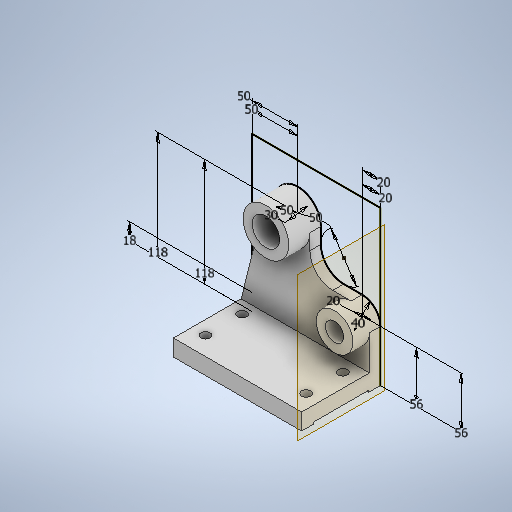
# Autodesk Inventor part: Baitap2
Saved by Autodesk Inventor 2025.2 (Build 292293000, 293)
## iProperties
Created: 2024-12-04
Part Number: Baitap2
Material: Generic
Document SubType Name: Modeling
Designer: hongquan
Density: 1 g/cm^3
Appearance: Default
Author: hongquan
Autodesk Inventor part; units mm, degrees
ref_plane "YZ Plane" through (0, 0, 0) normal (1, 0, 0) x (0, 1, 0)
ref_plane "XZ Plane" through (0, 0, 0) normal (0, 1, 0) x (-1, 0, 0)
ref_plane "XY Plane" through (0, 0, 0) normal (0, 0, 1) x (1, 0, 0)
sketch "Sketch1" plane through (0, 0, 0) normal (1, 0, 0) x (0, 1, 0)
  line L0 (0, 0) -> (168, 0)
  line L1 (168, 0) -> (168, -86)
  line L2 (168, -86) -> (0, -86)
  line L3 (0, -86) -> (0, 0)
  dimension "d0" = 86
  dimension "d1" = 168
  constraints: 8 end point, 2 parallel, 1 horizontal, 1 perpendicular
  measures "d0" distance of L2.end L0.start
  measures "d1" distance of L1.end L2.end
extrude "Extrusion1" add sketch "Sketch1" along normal blind 140
sketch "Sketch2" plane through (140, 0, 0) normal (1, 0, 0) x (0, 0, -1)
  line L0 (0, 0) -> (86, 0) projected
  line L1 (0, 0) -> (0, 2)
  line L2 (13, 2) -> (73, 2)
  line L3 (0, 168) -> (0, 0) projected
  line L4 (86, 168) -> (0, 168) projected
  line L5 (43, 168) -> (43, 0)
  line L6 (13, 2) -> (13, 0)
  line L7 (73, 2) -> (73, 0)
  line L8 (13, 0) -> (73, 0)
  point P0 (43, 2)
  dimension "d5" = 60
  dimension "d6" = 2
  constraints: 12 end point, 4 point on line, 3 midpoint, 2 collinear, 2 perpendicular, 1 horizontal, 1 vertical
  measures "d5" distance of L2.start L2.end
  measures "d6" distance from line of L0 L2.end
extrude "Extrusion2" cut sketch "Sketch2" against normal blind 140 contours L6 L2 L5 L0 | L5 L2 L7 L0
sketch "Sketch3" plane through (0, 0, -86) normal (0, 0, -1) x (-1, 0, 0)
  line L0 (-140, 0) -> (-140, 168) projected
  line L1 (-140, 0) -> (-140, 56)
  circle A0 centre (-120, 56) radius 10
  circle A1 centre (-120, 56) radius 20
  line L2 (0, 0) -> (-140, 0) projected
  circle A2 centre (-50, 118) radius 15
  circle A3 centre (-50, 118) radius 25
  line L3 (0, 0) -> (0, 168) projected
  arc A4 (-100, 76) -> (-75, 101) centre (-100, 101) ccw
  line L4 (0, 18) -> (0, 0)
  line L5 (-25, 118) -> (0, 18)
  line L6 (-75, 101) -> (-75, 118)
  line L7 (-100, 76) -> (-120, 76)
  line L8 (0, 168) -> (0, 18)
  line L9 (0, 168) -> (-140, 168) projected
  line L10 (0, 168) -> (-140, 168)
  line L11 (-140, 168) -> (-140, 56)
  dimension "d11" = 40
  dimension "d10" = 20
  dimension "d12" = 56
  dimension "d13" = 56
  dimension "d14" = 20
  dimension "d15" = 20
  dimension "d16" = 30
  dimension "d17" = 50
  dimension "d18" = 118
  dimension "d19" = 118
  dimension "d20" = 50
  dimension "d21" = 50
  dimension "d22" = 50
  dimension "d24" = 18
  constraints: 16 end point, 4 centre point, 4 point on circle, 3 horizontal, 3 tangent, 2 perpendicular, 2 point on line, 2 vertical, 1 collinear, 3 other
  measures "d10" diameter of A0
  measures "d12" distance from line of L2 point (-120, 56)
  measures "d13" distance from line of L2 A0.centre
  measures "d14" distance from line of L0 A0.centre
  measures "d15" distance from line of L0 point (-120, 56)
  measures "d16" diameter of A2
  measures "d17" diameter of A3
  measures "d18" distance from line of L2 A3.centre
  measures "d19" distance from line of L2 A2.centre
  measures "d20" distance from line of L3 A3.centre
  measures "d21" distance from line of L3 A2.centre
  measures "d22" diameter of A4
  measures "d24" distance of L2.start L4.start
extrude "Extrusion3" cut sketch "Sketch3" against normal blind 140 contours L0 L9 L3 L5 A3 L6 A4 L7 A1 | A0 | A2
ref_plane "Work Plane1" through (140, 28, 0) normal (1, 0, 0) x (0, 0, -1)
sketch "Sketch4" plane through (140, 28, 0) normal (1, 0, 0) x (0, 0, -1)
  line L0 (73, -28) -> (86, -28) projected
  line L1 (86, -28) -> (86, -10) projected
  line L2 (86, -28) -> (86, -10)
  line L3 (86, -10) -> (0, -10)
  line L4 (0, -10) -> (0, -28)
  line L5 (86, 90) -> (86, 115) projected
  line L6 (0, 115) -> (0, 90) projected
  line L7 (86, 115) -> (0, 115)
  line L8 (86, 115) -> (74, 115)
  line L9 (74, 115) -> (74, -10)
  line L10 (0, 90) -> (0, -10) projected
  line L11 (0, -10) -> (0, 115)
  dimension "d29" = 12
  constraints: 14 end point, 3 perpendicular, 2 point on line, 1 collinear, 1 horizontal, 1 vertical
  measures "d29" distance of L5.end L8.end
extrude "Extrusion4" cut sketch "Sketch4" against normal blind 140
extrude "Extrusion5" add sketch "Sketch3" against normal blind 35 contours A3
extrude "Extrusion6" add sketch "Sketch3" against normal blind 30 contours A1 | A0
extrude "Extrusion7" cut sketch "Sketch3" against normal blind 30 contours A0
sketch "Sketch5" plane through (140, 2, -73) normal (0, -1, 0) x (1, 0, 0)
  circle A0 centre (-15, 53) radius 5
  line L0 (-140, 73) -> (0, 73) projected
  line L1 (0, 60) -> (0, 0) projected
  circle A1 centre (-125, 53) radius 5
  circle A2 centre (-125, 13) radius 5
  circle A3 centre (-15, 13) radius 5
  dimension "d38" = 10
  dimension "d39" = 20
  dimension "d40" = 15
  dimension "d41" = 10
  dimension "d42" = 110
  dimension "d43" = 20
  dimension "d44" = 10
  dimension "d45" = 40
  dimension "d46" = 125
  dimension "d47" = 10
  dimension "d48" = 15
  dimension "d49" = 40
  constraints: 4 centre point
  measures "d38" diameter of A0
  measures "d39" distance from line of L0 A0.centre
  measures "d40" distance from line of L1 A0.centre
  measures "d41" diameter of A1
  measures "d42" distance of A1.centre A0.centre
  measures "d43" distance from line of L0 A1.centre
  measures "d44" diameter of A2
  measures "d45" distance of A1.centre A2.centre
  measures "d46" distance from line of L1 A2.centre
  measures "d47" diameter of A3
  measures "d48" distance from line of L1 A3.centre
  measures "d49" distance of A0.centre A3.centre
extrude "Extrusion8" cut sketch "Sketch5" against normal blind 30
body "Solid1"
